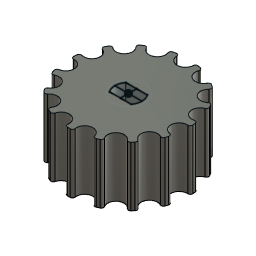
timingBeltGearStepper (Autodesk Fusion 360 design; units mm, degrees)
Autodesk Fusion 360 part; units mm, degrees
sketch "Sketch1" plane through (0, 0, 0) normal (0, 1, 0) x (1, 0, 0)
  circle A0 centre (0, 0) radius 11.0666 construction
  circle A1 centre (0, 0) radius 9.0066 construction
  line L0 (0, 0) -> (0, 11.0666) construction
  line L1 (0, 0) -> (4.5012, 10.1099) construction
  line L2 (0, 0) -> (39.7887, 0) construction
  arc A2 (2.6812, 10.7198) -> (2.5679, 10.7646) centre (2.4681, 10.3463) ccw
  line L3 (2.043, 10.8763) -> (2.5679, 10.7646)
  arc A3 (0, 9.0066) -> (1.5238, 10.4724) centre (0, 10.5316) ccw
  arc A4 (2.8674, 10.1868) -> (2.5679, 10.7646) centre (2.4681, 10.3463) ccw
  arc A5 (2.043, 10.8763) -> (1.5238, 10.4724) centre (1.9535, 10.4557) ccw
  arc A6 (2.8674, 10.1868) -> (3.6633, 8.228) centre (4.2836, 9.6211) ccw
  arc A7 (-3.6633, 8.228) -> (-2.8674, 10.1868) centre (-4.2836, 9.6211) ccw
  arc A8 (-2.5574, 10.7669) -> (-2.8674, 10.1868) centre (-2.4681, 10.3463) ccw
  line L4 (-2.5574, 10.7669) -> (-2.0325, 10.8784)
  arc A9 (-1.5238, 10.4724) -> (-2.0325, 10.8784) centre (-1.9535, 10.4557) ccw
  arc A10 (-1.5238, 10.4724) -> (0, 9.0066) centre (0, 10.5316) ccw
  arc A11 (-6.6932, 6.0266) -> (-6.7628, 8.1398) centre (-7.8265, 7.047) ccw
  arc A12 (-6.7156, 8.7959) -> (-6.7628, 8.1398) centre (-6.4629, 8.448) ccw
  line L5 (-6.7156, 8.7959) -> (-6.2814, 9.1112)
  arc A13 (-5.6516, 8.9472) -> (-6.2814, 9.1112) centre (-6.0373, 8.7572) ccw
  arc A14 (-5.6516, 8.9472) -> (-3.6633, 8.228) centre (-4.2836, 9.6211) ccw
  arc A15 (-8.5658, 2.7832) -> (-9.4889, 4.6854) centre (-10.0162, 3.2544) ccw
  arc A16 (-9.7126, 5.304) -> (-9.4889, 4.6854) centre (-9.3403, 5.0889) ccw
  line L6 (-9.7126, 5.304) -> (-9.4442, 5.7686)
  arc A17 (-8.8022, 5.875) -> (-9.4442, 5.7686) centre (-9.0773, 5.5445) ccw
  arc A18 (-8.8022, 5.875) -> (-6.6932, 6.0266) centre (-7.8265, 7.047) ccw
  arc A19 (-8.9573, -0.9414) -> (-10.5743, 0.4208) centre (-10.4739, -1.1009) ccw
  arc A20 (-11.0302, 0.895) -> (-10.5743, 0.4208) centre (-10.6026, 0.8499) ccw
  line L7 (-11.0302, 0.895) -> (-10.974, 1.4286)
  arc A21 (-10.4307, 1.7869) -> (-10.974, 1.4286) centre (-10.5476, 1.3731) ccw
  arc A22 (-10.4307, 1.7869) -> (-8.5658, 2.7832) centre (-10.0162, 3.2544) ccw
  arc A23 (-7.8, -4.5033) -> (-9.8313, -3.9165) centre (-9.1207, -5.2658) ccw
  arc A24 (-10.4406, -3.6688) -> (-9.8313, -3.9165) centre (-10.0317, -3.536) ccw
  line L8 (-10.4406, -3.6688) -> (-10.6063, -3.1585)
  arc A25 (-10.2557, -2.6102) -> (-10.6063, -3.1585) centre (-10.1942, -3.0357) ccw
  arc A26 (-10.2557, -2.6102) -> (-8.9573, -0.9414) centre (-10.4739, -1.1009) ccw
  arc A27 (-5.294, -7.2865) -> (-7.3883, -7.5766) centre (-6.1903, -8.5203) ccw
  arc A28 (-8.0458, -7.5982) -> (-7.3883, -7.5766) centre (-7.7261, -7.3106) ccw
  line L9 (-8.0458, -7.5982) -> (-8.4047, -7.1994)
  arc A29 (-8.3074, -6.5559) -> (-8.4047, -7.1994) centre (-8.0781, -6.9196) ccw
  arc A30 (-8.3074, -6.5559) -> (-7.8, -4.5033) centre (-9.1207, -5.2658) ccw
  arc A31 (-1.8726, -8.8098) -> (-3.6679, -9.9267) centre (-2.1896, -10.3015) ccw
  arc A32 (-4.2597, -10.2138) -> (-3.6679, -9.9267) centre (-4.0847, -9.821) ccw
  line L10 (-4.2597, -10.2138) -> (-4.7498, -9.9955)
  arc A33 (-4.9227, -9.368) -> (-4.7498, -9.9955) centre (-4.5653, -9.6071) ccw
  arc A34 (-4.9227, -9.368) -> (-5.294, -7.2865) centre (-6.1903, -8.5203) ccw
  arc A35 (1.8726, -8.8098) -> (0.6868, -10.5604) centre (2.1896, -10.3015) ccw
  arc A36 (0.2629, -11.0634) -> (0.6868, -10.5604) centre (0.263, -10.6334) ccw
  line L11 (0.2629, -11.0634) -> (-0.2737, -11.0632)
  arc A37 (-0.6868, -10.5604) -> (-0.2737, -11.0632) centre (-0.263, -10.6334) ccw
  arc A38 (-0.6868, -10.5604) -> (-1.8726, -8.8098) centre (-2.1896, -10.3015) ccw
  arc A39 (5.294, -7.2865) -> (4.9227, -9.368) centre (6.1903, -8.5203) ccw
  arc A40 (4.7401, -10) -> (4.9227, -9.368) centre (4.5653, -9.6071) ccw
  line L12 (4.7401, -10) -> (4.2498, -10.2181)
  arc A41 (3.6679, -9.9267) -> (4.2498, -10.2181) centre (4.0847, -9.821) ccw
  arc A42 (3.6679, -9.9267) -> (1.8726, -8.8098) centre (2.1896, -10.3015) ccw
  arc A43 (7.8, -4.5033) -> (8.3074, -6.5559) centre (9.1207, -5.2658) ccw
  arc A44 (8.3976, -7.2075) -> (8.3074, -6.5559) centre (8.0781, -6.9196) ccw
  line L13 (8.3976, -7.2075) -> (8.0385, -7.6061)
  arc A45 (7.3883, -7.5766) -> (8.0385, -7.6061) centre (7.7261, -7.3106) ccw
  arc A46 (7.3883, -7.5766) -> (5.294, -7.2865) centre (6.1903, -8.5203) ccw
  arc A47 (8.9573, -0.9414) -> (10.2557, -2.6102) centre (10.4739, -1.1009) ccw
  arc A48 (10.6031, -3.1687) -> (10.2557, -2.6102) centre (10.1942, -3.0357) ccw
  line L14 (10.6031, -3.1687) -> (10.4372, -3.679)
  arc A49 (9.8313, -3.9165) -> (10.4372, -3.679) centre (10.0317, -3.536) ccw
  arc A50 (9.8313, -3.9165) -> (7.8, -4.5033) centre (9.1207, -5.2658) ccw
  arc A51 (8.5658, 2.7832) -> (10.4307, 1.7869) centre (10.0162, 3.2544) ccw
  arc A52 (10.9753, 1.4179) -> (10.4307, 1.7869) centre (10.5476, 1.3731) ccw
  line L15 (10.9753, 1.4179) -> (11.0312, 0.8843)
  arc A53 (10.5743, 0.4208) -> (11.0312, 0.8843) centre (10.6026, 0.8499) ccw
  arc A54 (10.5743, 0.4208) -> (8.9573, -0.9414) centre (10.4739, -1.1009) ccw
  arc A55 (6.6932, 6.0266) -> (8.8022, 5.875) centre (7.8265, 7.047) ccw
  arc A56 (9.4497, 5.7594) -> (8.8022, 5.875) centre (9.0773, 5.5445) ccw
  line L16 (9.4497, 5.7594) -> (9.7179, 5.2946)
  arc A57 (9.4889, 4.6854) -> (9.7179, 5.2946) centre (9.3403, 5.0889) ccw
  arc A58 (9.4889, 4.6854) -> (8.5658, 2.7832) centre (10.0162, 3.2544) ccw
  arc A59 (3.6633, 8.228) -> (5.6516, 8.9472) centre (4.2836, 9.6211) ccw
  arc A60 (6.2902, 9.105) -> (5.6516, 8.9472) centre (6.0373, 8.7572) ccw
  line L17 (6.2902, 9.105) -> (6.7242, 8.7895)
  arc A61 (6.7628, 8.1398) -> (6.7242, 8.7895) centre (6.4629, 8.448) ccw
  arc A62 (6.7628, 8.1398) -> (6.6932, 6.0266) centre (7.8265, 7.047) ccw
  dimension "d25" = 22.1332
  dimension "d26" = 18.0132
  dimension "d27" = 11.0666
  dimension "d28" = 66
  dimension "d29" = 11.0666
  dimension "d31" = 3.05
  dimension "d32" = 3.05
  dimension "d33" = 0.86
  dimension "d34" = 0.86
  dimension "d36" = 360
  constraint coincident A0.centre A1.centre
  constraint vertical L0
  constraint horizontal L2
  constraint coincident L0 A3.centre
  constraint tangent A1 A3
  constraint coincident L1 A6.centre
  constraint tangent A1 A6
  constraint tangent A4 A6
  constraint tangent A0 A4
  constraint tangent A3 A5
  constraint tangent A0 A5
  constraint coincident A0 A2.end
  constraint coincident A2.end A4
  constraint coincident A2.start A4
  constraint coincident A2.centre A4.centre
  constraint tangent L3 A5
  constraint coincident A1 A3.start
  constraint coincident A1 A6.end
  measures "d25" diameter of A0
  measures "d26" diameter of A1
  measures "d27" distance of A0.centre L0.end
  measures "d28" angle of L1 L2
  measures "d29" distance of A0.centre L1.end
  measures "d31" diameter of A3
  measures "d32" diameter of A6
  measures "d33" diameter of A5
  measures "d34" diameter of A4
extrude "Extrude2" add sketch "Sketch1" along normal blind 11
sketch "Sketch2" plane through (0, 11, 0) normal (0, 1, 0) x (-1, 0, 0)
  arc A0 (-2.8674, -10.1868) -> (-5.6516, -8.9472) centre (-4.2836, -9.6211) ccw
  arc A1 (-2.8674, -10.1868) -> (-2.5679, -10.7646) centre (-2.4681, -10.3463) ccw
  line L0 (-2.5679, -10.7646) -> (-2.043, -10.8763)
  arc A2 (-2.043, -10.8763) -> (-1.5238, -10.4724) centre (-1.9535, -10.4557) ccw
  arc A3 (1.5238, -10.4724) -> (-1.5238, -10.4724) centre (0, -10.5316) ccw
  arc A4 (1.5238, -10.4724) -> (2.0325, -10.8784) centre (1.9535, -10.4557) ccw
  line L1 (2.0325, -10.8784) -> (2.5574, -10.7669)
  arc A5 (2.5574, -10.7669) -> (2.8674, -10.1868) centre (2.4681, -10.3463) ccw
  arc A6 (5.6516, -8.9472) -> (2.8674, -10.1868) centre (4.2836, -9.6211) ccw
  arc A7 (5.6516, -8.9472) -> (6.2814, -9.1112) centre (6.0373, -8.7572) ccw
  line L2 (6.2814, -9.1112) -> (6.7156, -8.7959)
  arc A8 (6.7156, -8.7959) -> (6.7628, -8.1398) centre (6.4629, -8.448) ccw
  arc A9 (8.8022, -5.875) -> (6.7628, -8.1398) centre (7.8265, -7.047) ccw
  arc A10 (8.8022, -5.875) -> (9.4442, -5.7686) centre (9.0773, -5.5445) ccw
  line L3 (9.4442, -5.7686) -> (9.7126, -5.304)
  arc A11 (9.7126, -5.304) -> (9.4889, -4.6854) centre (9.3403, -5.0889) ccw
  arc A12 (10.4307, -1.7869) -> (9.4889, -4.6854) centre (10.0162, -3.2544) ccw
  arc A13 (10.4307, -1.7869) -> (10.974, -1.4286) centre (10.5476, -1.3731) ccw
  line L4 (10.974, -1.4286) -> (11.0302, -0.895)
  arc A14 (11.0302, -0.895) -> (10.5743, -0.4208) centre (10.6026, -0.8499) ccw
  arc A15 (10.2557, 2.6102) -> (10.5743, -0.4208) centre (10.4739, 1.1009) ccw
  arc A16 (10.2557, 2.6102) -> (10.6063, 3.1585) centre (10.1942, 3.0357) ccw
  line L5 (10.6063, 3.1585) -> (10.4406, 3.6688)
  arc A17 (10.4406, 3.6688) -> (9.8313, 3.9165) centre (10.0317, 3.536) ccw
  arc A18 (8.3074, 6.5559) -> (9.8313, 3.9165) centre (9.1207, 5.2658) ccw
  arc A19 (8.3074, 6.5559) -> (8.4047, 7.1994) centre (8.0781, 6.9196) ccw
  line L6 (8.4047, 7.1994) -> (8.0458, 7.5982)
  arc A20 (8.0458, 7.5982) -> (7.3883, 7.5766) centre (7.7261, 7.3106) ccw
  arc A21 (4.9227, 9.368) -> (7.3883, 7.5766) centre (6.1903, 8.5203) ccw
  arc A22 (4.9227, 9.368) -> (4.7498, 9.9955) centre (4.5653, 9.6071) ccw
  line L7 (4.7498, 9.9955) -> (4.2597, 10.2138)
  arc A23 (4.2597, 10.2138) -> (3.6679, 9.9267) centre (4.0847, 9.821) ccw
  arc A24 (0.6868, 10.5604) -> (3.6679, 9.9267) centre (2.1896, 10.3015) ccw
  arc A25 (0.6868, 10.5604) -> (0.2737, 11.0632) centre (0.263, 10.6334) ccw
  line L8 (0.2737, 11.0632) -> (-0.2629, 11.0634)
  arc A26 (-0.2629, 11.0634) -> (-0.6868, 10.5604) centre (-0.263, 10.6334) ccw
  arc A27 (-3.6679, 9.9267) -> (-0.6868, 10.5604) centre (-2.1896, 10.3015) ccw
  arc A28 (-3.6679, 9.9267) -> (-4.2498, 10.2181) centre (-4.0847, 9.821) ccw
  line L9 (-4.2498, 10.2181) -> (-4.7401, 10)
  arc A29 (-4.7401, 10) -> (-4.9227, 9.368) centre (-4.5653, 9.6071) ccw
  arc A30 (-7.3883, 7.5766) -> (-4.9227, 9.368) centre (-6.1903, 8.5203) ccw
  arc A31 (-7.3883, 7.5766) -> (-8.0385, 7.6061) centre (-7.7261, 7.3106) ccw
  line L10 (-8.0385, 7.6061) -> (-8.3976, 7.2075)
  arc A32 (-8.3976, 7.2075) -> (-8.3074, 6.5559) centre (-8.0781, 6.9196) ccw
  arc A33 (-9.8313, 3.9165) -> (-8.3074, 6.5559) centre (-9.1207, 5.2658) ccw
  arc A34 (-9.8313, 3.9165) -> (-10.4372, 3.679) centre (-10.0317, 3.536) ccw
  line L11 (-10.4372, 3.679) -> (-10.6031, 3.1687)
  arc A35 (-10.6031, 3.1687) -> (-10.2557, 2.6102) centre (-10.1942, 3.0357) ccw
  arc A36 (-10.5743, -0.4208) -> (-10.2557, 2.6102) centre (-10.4739, 1.1009) ccw
  arc A37 (-10.5743, -0.4208) -> (-11.0312, -0.8843) centre (-10.6026, -0.8499) ccw
  line L12 (-11.0312, -0.8843) -> (-10.9753, -1.4179)
  arc A38 (-10.9753, -1.4179) -> (-10.4307, -1.7869) centre (-10.5476, -1.3731) ccw
  arc A39 (-9.4889, -4.6854) -> (-10.4307, -1.7869) centre (-10.0162, -3.2544) ccw
  arc A40 (-9.4889, -4.6854) -> (-9.7179, -5.2946) centre (-9.3403, -5.0889) ccw
  line L13 (-9.7179, -5.2946) -> (-9.4497, -5.7594)
  arc A41 (-9.4497, -5.7594) -> (-8.8022, -5.875) centre (-9.0773, -5.5445) ccw
  arc A42 (-6.7628, -8.1398) -> (-8.8022, -5.875) centre (-7.8265, -7.047) ccw
  arc A43 (-6.7628, -8.1398) -> (-6.7242, -8.7895) centre (-6.4629, -8.448) ccw
  line L14 (-6.7242, -8.7895) -> (-6.2902, -9.105)
  arc A44 (-6.2902, -9.105) -> (-5.6516, -8.9472) centre (-6.0373, -8.7572) ccw
  circle A45 centre (0, 0) radius 3
  circle A46 centre (0, 0) radius 12.5
  dimension "d39" = 6
  dimension "d40" = 25
  constraint coincident A45.centre A46.centre
  measures "d39" diameter of A45
  measures "d40" diameter of A46
extrude "Extrude7" cut sketch "Sketch2" against normal blind 13 contours A45
sketch "Sketch3" plane through (0, 11, 0) normal (0, 1, 0) x (-1, 0, 0)
  circle A0 centre (0, 0) radius 3
  arc A1 (-6.2902, -9.105) -> (-5.6516, -8.9472) centre (-6.0373, -8.7572) ccw
  arc A2 (-2.8674, -10.1868) -> (-5.6516, -8.9472) centre (-4.2836, -9.6211) ccw
  arc A3 (-2.8674, -10.1868) -> (-2.5679, -10.7646) centre (-2.4681, -10.3463) ccw
  line L0 (-2.5679, -10.7646) -> (-2.043, -10.8763)
  arc A4 (-2.043, -10.8763) -> (-1.5238, -10.4724) centre (-1.9535, -10.4557) ccw
  arc A5 (1.5238, -10.4724) -> (-1.5238, -10.4724) centre (0, -10.5316) ccw
  arc A6 (1.5238, -10.4724) -> (2.0325, -10.8784) centre (1.9535, -10.4557) ccw
  line L1 (2.0325, -10.8784) -> (2.5574, -10.7669)
  arc A7 (2.5574, -10.7669) -> (2.8674, -10.1868) centre (2.4681, -10.3463) ccw
  arc A8 (5.6516, -8.9472) -> (2.8674, -10.1868) centre (4.2836, -9.6211) ccw
  arc A9 (5.6516, -8.9472) -> (6.2814, -9.1112) centre (6.0373, -8.7572) ccw
  line L2 (6.2814, -9.1112) -> (6.7156, -8.7959)
  arc A10 (6.7156, -8.7959) -> (6.7628, -8.1398) centre (6.4629, -8.448) ccw
  arc A11 (8.8022, -5.875) -> (6.7628, -8.1398) centre (7.8265, -7.047) ccw
  arc A12 (8.8022, -5.875) -> (9.4442, -5.7686) centre (9.0773, -5.5445) ccw
  line L3 (9.4442, -5.7686) -> (9.7126, -5.304)
  arc A13 (9.7126, -5.304) -> (9.4889, -4.6854) centre (9.3403, -5.0889) ccw
  arc A14 (10.4307, -1.7869) -> (9.4889, -4.6854) centre (10.0162, -3.2544) ccw
  arc A15 (10.4307, -1.7869) -> (10.974, -1.4286) centre (10.5476, -1.3731) ccw
  line L4 (10.974, -1.4286) -> (11.0302, -0.895)
  arc A16 (11.0302, -0.895) -> (10.5743, -0.4208) centre (10.6026, -0.8499) ccw
  arc A17 (10.2557, 2.6102) -> (10.5743, -0.4208) centre (10.4739, 1.1009) ccw
  arc A18 (10.2557, 2.6102) -> (10.6063, 3.1585) centre (10.1942, 3.0357) ccw
  line L5 (10.6063, 3.1585) -> (10.4406, 3.6688)
  arc A19 (10.4406, 3.6688) -> (9.8313, 3.9165) centre (10.0317, 3.536) ccw
  arc A20 (8.3074, 6.5559) -> (9.8313, 3.9165) centre (9.1207, 5.2658) ccw
  arc A21 (8.3074, 6.5559) -> (8.4047, 7.1994) centre (8.0781, 6.9196) ccw
  line L6 (8.4047, 7.1994) -> (8.0458, 7.5982)
  arc A22 (8.0458, 7.5982) -> (7.3883, 7.5766) centre (7.7261, 7.3106) ccw
  arc A23 (4.9227, 9.368) -> (7.3883, 7.5766) centre (6.1903, 8.5203) ccw
  arc A24 (4.9227, 9.368) -> (4.7498, 9.9955) centre (4.5653, 9.6071) ccw
  line L7 (4.7498, 9.9955) -> (4.2597, 10.2138)
  arc A25 (4.2597, 10.2138) -> (3.6679, 9.9267) centre (4.0847, 9.821) ccw
  arc A26 (0.6868, 10.5604) -> (3.6679, 9.9267) centre (2.1896, 10.3015) ccw
  arc A27 (0.6868, 10.5604) -> (0.2737, 11.0632) centre (0.263, 10.6334) ccw
  line L8 (0.2737, 11.0632) -> (-0.2629, 11.0634)
  arc A28 (-0.2629, 11.0634) -> (-0.6868, 10.5604) centre (-0.263, 10.6334) ccw
  arc A29 (-3.6679, 9.9267) -> (-0.6868, 10.5604) centre (-2.1896, 10.3015) ccw
  arc A30 (-3.6679, 9.9267) -> (-4.2498, 10.2181) centre (-4.0847, 9.821) ccw
  line L9 (-4.2498, 10.2181) -> (-4.7401, 10)
  arc A31 (-4.7401, 10) -> (-4.9227, 9.368) centre (-4.5653, 9.6071) ccw
  arc A32 (-7.3883, 7.5766) -> (-4.9227, 9.368) centre (-6.1903, 8.5203) ccw
  arc A33 (-7.3883, 7.5766) -> (-8.0385, 7.6061) centre (-7.7261, 7.3106) ccw
  line L10 (-8.0385, 7.6061) -> (-8.3976, 7.2075)
  arc A34 (-8.3976, 7.2075) -> (-8.3074, 6.5559) centre (-8.0781, 6.9196) ccw
  arc A35 (-9.8313, 3.9165) -> (-8.3074, 6.5559) centre (-9.1207, 5.2658) ccw
  arc A36 (-9.8313, 3.9165) -> (-10.4372, 3.679) centre (-10.0317, 3.536) ccw
  line L11 (-10.4372, 3.679) -> (-10.6031, 3.1687)
  arc A37 (-10.6031, 3.1687) -> (-10.2557, 2.6102) centre (-10.1942, 3.0357) ccw
  arc A38 (-10.5743, -0.4208) -> (-10.2557, 2.6102) centre (-10.4739, 1.1009) ccw
  arc A39 (-10.5743, -0.4208) -> (-11.0312, -0.8843) centre (-10.6026, -0.8499) ccw
  line L12 (-11.0312, -0.8843) -> (-10.9753, -1.4179)
  arc A40 (-10.9753, -1.4179) -> (-10.4307, -1.7869) centre (-10.5476, -1.3731) ccw
  arc A41 (-9.4889, -4.6854) -> (-10.4307, -1.7869) centre (-10.0162, -3.2544) ccw
  arc A42 (-9.4889, -4.6854) -> (-9.7179, -5.2946) centre (-9.3403, -5.0889) ccw
  line L13 (-9.7179, -5.2946) -> (-9.4497, -5.7594)
  arc A43 (-9.4497, -5.7594) -> (-8.8022, -5.875) centre (-9.0773, -5.5445) ccw
  arc A44 (-6.7628, -8.1398) -> (-8.8022, -5.875) centre (-7.8265, -7.047) ccw
  arc A45 (-6.7628, -8.1398) -> (-6.7242, -8.7895) centre (-6.4629, -8.448) ccw
  line L14 (-6.7242, -8.7895) -> (-6.2902, -9.105)
  line L15 (0, 0) -> (0, -1.5)
  line L16 (0, 0) -> (0, 1.5)
  line L17 (0, 0) -> (2.5, 0)
  line L18 (0, 0) -> (-2.5, 0)
  line L19 (0, 1.5) -> (2, 1.5)
  line L20 (0, 1.5) -> (-2, 1.5)
  line L21 (0, -1.5) -> (2, -1.5)
  line L22 (0, -1.5) -> (-2, -1.5)
  arc A46 (-2, 1.5) -> (-2, -1.5) centre (0, 0) ccw
  arc A47 (2, -1.5) -> (2, 1.5) centre (0, 0) ccw
  dimension "d52" = 1.5
  dimension "d53" = 1.5
  dimension "d54" = 2.5
  dimension "d55" = 2.5
  dimension "d56" = 2
  dimension "d57" = 2
  dimension "d58" = 2
  dimension "d59" = 2
  constraint coincident A0.centre L15.start
  constraint vertical L15
  constraint parallel L15 L16
  constraint perpendicular L16 L17
  constraint perpendicular L16 L18
  constraint perpendicular L16 L19
  constraint perpendicular L16 L20
  constraint perpendicular L15 L21
  constraint perpendicular L15 L22
  constraint coincident L18.end A46
  constraint coincident L17.end A47
  measures "d52" distance of A0.centre L15.end
  measures "d53" distance of A0.centre L16.end
  measures "d54" distance of A0.centre L17.end
  measures "d55" distance of A0.centre L18.end
  measures "d56" distance of L16.end L19.end
  measures "d57" distance of L16.end L20.end
  measures "d58" distance of L15.end L21.end
  measures "d59" distance of L15.end L22.end
extrude "Extrude8" add sketch "Sketch3" against normal blind 11 contours A0
equation "outerCircleDia = ( ( ( 5 * numTeeth ) / PI ) * 1 mm ) - ( 3.8 mm - 2.06 mm )" comment "HTD5 - Outer circle diameter. (5mm spacing * number of teeth) - bend point of belt*2 - Equation based on Circumference = 2*Pi*r. Belt bent point will effectively compress the teeth together, making spacing less than 5mm, therefore the diameter is adjusted with the assumed bend point. effectively this is likely to be closer to the teeth than the outside of the belt due to the kevlar beeing closer to the inside."
equation "innerCircleDia = outerCircleDia - ( 2.06 ) * 2 * 1 mm" comment "HTD5 - outer circle diameter minus 2 times height of tooth."
equation "numTeeth = 15" comment "HTD5 - Number of teeth."
equation "toothAngle = ( 360 / numTeeth ) * 1 deg" comment "HTD5 - Degrees between teeth. full rotation divided by number of teeth per rotation."
equation "Width = 11 mm" comment "HTD5 - Width"
equation "d25 = outerCircleDia"
equation "d26 = innerCircleDia"
equation "d27 = outerCircleDia / 2"
equation "d28 = 90 deg - toothAngle"
equation "d29 = outerCircleDia / 2"
equation "d35 = numTeeth"
equation "d37 = Width"
